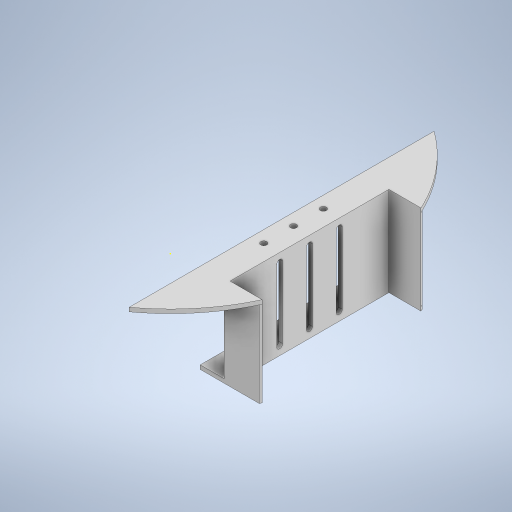
# Autodesk Inventor part: Base-Dribler
Saved by Autodesk Inventor 2024.2 (Build 282272000, 272)
## iProperties
Created: 2023-12-01
Part Number: Base-Dribler
Material: Generic
Document SubType Name: Modeling
Designer: felip
Density: 1 g/cm^3
Appearance: Default
Author: felip
Autodesk Inventor part; units mm, degrees
ref_plane "YZ Plane" through (0, 0, 0) normal (1, 0, 0) x (0, 1, 0)
ref_plane "XZ Plane" through (0, 0, 0) normal (0, 1, 0) x (-1, 0, 0)
ref_plane "XY Plane" through (0, 0, 0) normal (0, 0, 1) x (1, 0, 0)
sketch "Sketch3" plane through (0, 0, 0) normal (0, 1, 0) x (-1, 0, 0)
  circle A0 centre (0, 0) radius 95
  line L0 (-68, 0) -> (-68, -40)
  line L1 (-68, 0) -> (-68, 40)
  line L2 (-68, 40) -> (-86.1684, 40)
  line L3 (-68, -40) -> (-86.1684, -40)
  line L4 (-56, 0) -> (-56, -76.7398)
  line L5 (-56, 0) -> (-56, 76.7398)
  line L6 (-62, 0) -> (-62, -15)
  line L7 (-62, 0) -> (-62, 15)
  circle A1 centre (-62, 15) radius 1.5
  circle A2 centre (-62, 0) radius 1.5
  circle A3 centre (-62, -15) radius 1.5
  line L8 (-68, 0) -> (-70, 0)
  line L9 (-70, 0) -> (-70, -40)
  line L10 (-70, 0) -> (-70, 40)
  dimension "d1" = 68
  dimension "d2" = 40
  dimension "d3" = 40
  dimension "d4" = 12
  dimension "d5" = 6
  dimension "d6" = 15
  dimension "d7" = 15
  dimension "d8" = 3
  dimension "d9" = 3
  dimension "d10" = 3
  dimension "d11" = 2
  constraints: 22 end point, 4 centre point, 4 coincident, 4 point on circle, 4 point on line, 3 vertical, 2 perpendicular, 1 horizontal, 1 parallel
  measures "d1" distance of A0.centre L0.start
  measures "d2" distance of L0.start L0.end
  measures "d3" distance of L0.start L1.end
  measures "d4" distance of L0.start L4.start
  measures "d5" distance of L0.start L6.start
  measures "d6" distance of L6.start L6.end
  measures "d7" distance of L6.start L7.end
  measures "d8" diameter of A1
  measures "d9" diameter of A2
  measures "d10" diameter of A3
  measures "d11" distance of L0.start L8.end
extrude "Extrusion1" add sketch "Sketch3" along normal blind 2 contours L5 L4 A0 L3 L0 L1 L2 | L2 L1 L8 L10 | L9 L8 L0 L3
sketch "Sketch4" plane through (0, 0, 0) normal (0, -1, 0) x (1, 0, 0)
  line L0 (70, 40) -> (70, -40) projected
  line L1 (70, 0) -> (68, 0)
  line L2 (68, 0) -> (68, -40)
  line L3 (70, -41) -> (85.6971, -41)
  arc A0 (56, -76.7398) -> (86.1684, -40) centre (0, 0) ccw projected
  line L4 (68, -40) -> (68, -41)
  line L5 (70, -41) -> (68, -41)
  line L6 (85.6971, -41) -> (86.1684, -40)
  line L7 (70, -40) -> (86.1684, -40) projected
  line L8 (70, -40) -> (86.1684, -40)
  line L9 (70, -40) -> (70, 40)
  line L10 (86.1684, 40) -> (70, 40) projected
  line L11 (86.1684, 40) -> (70, 40)
  line L12 (68, 0) -> (68, 40)
  line L13 (70, 41) -> (85.6971, 41)
  arc A1 (86.1684, 40) -> (56, 76.7398) centre (0, 0) ccw projected
  line L14 (70, 41) -> (68, 41)
  line L15 (68, 40) -> (68, 41)
  line L16 (85.6971, 41) -> (86.1684, 40)
  dimension "d14" = 2
  dimension "d15" = 1
  constraints: 28 end point, 4 point on line, 3 horizontal, 3 perpendicular, 2 point on circle, 1 collinear, 1 midpoint, 1 vertical
  measures "d14" distance of L1.start L1.end
  measures "d15" distance of L0.end L3.start
extrude "Extrusion2" add sketch "Sketch4" along normal blind 41
sketch "Sketch5" plane through (0, -41, 0) normal (0, -1, 0) x (1, 0, 0)
  point P0 (0, 0)
sketch "Sketch6" plane through (0, -41, 0) normal (0, -1, 0) x (1, 0, 0)
  circle A0 centre (62, 15) radius 1.5 projected
  circle A1 centre (62, 15) radius 1.5
  circle A2 centre (62, 0) radius 1.5
  circle A3 centre (62, -15) radius 1.5 projected
  circle A4 centre (62, -15) radius 1.5
  line L0 (70, 40) -> (56, 40)
  line L1 (70, -40) -> (86.1684, -40) projected
  line L2 (70, -40) -> (56, -40)
  line L3 (56, -40) -> (56, 40)
  line L4 (70, 40) -> (70, -40) projected
  line L5 (70, 40) -> (70, -40)
  line L6 (86.1684, 40) -> (70, 40) projected
  line L7 (86.1684, 40) -> (70, 40)
  line L8 (70, -40) -> (86.1684, -40)
  line L9 (86.1684, 40) -> (85.6971, 41)
  arc A5 (86.1684, 40) -> (85.6971, 41) centre (0, 0) ccw projected
  line L10 (56, 40) -> (56, 41)
  line L11 (85.6971, 41) -> (56, 41)
  line L12 (56, -40) -> (56, -41)
  line L13 (86.1684, -40) -> (85.9357, -40.5014)
  line L14 (85.6971, -41) -> (56, -41)
  line L15 (85.9357, -40.5014) -> (85.6971, -41)
  arc A6 (56, -76.7398) -> (86.1684, -40) centre (0, 0) ccw projected
  constraints: 26 end point, 3 centre point, 3 horizontal, 3 perpendicular, 2 coincident, 2 collinear, 2 other
extrude "Extrusion3" add sketch "Sketch6" along normal blind 2 contours L4 L2 L3 L0
extrude "Extrusion5" add sketch "Sketch6" along normal blind 2 contours L0 L10 L11 L9 L6 | L1 L13 L15 L14 L12 L2
sketch "Sketch7" plane through (70, 2, 40) normal (1, 0, 0) x (0, 0, -1)
  line L0 (0, -2) -> (0, -45) projected
  line L1 (80, -2) -> (80, -43) projected
  line L2 (80, -22.5) -> (55, -22.5)
  line L3 (55, -22.5) -> (40, -22.5)
  line L4 (40, -22.5) -> (40, -4.5)
  line L5 (40, -22.5) -> (40, -40.5)
  line L6 (55, -22.5) -> (55, -4.5)
  line L7 (55, -22.5) -> (55, -40.5)
  line L8 (0, 0) -> (80, 0) projected
  line L9 (0, -22.5) -> (25, -22.5)
  line L10 (25, -22.5) -> (25, -4.5)
  line L11 (25, -22.5) -> (25, -40.5)
  line L12 (25, -4.5) -> (25, -40.5) construction
  line L13 (23.5, -4.5) -> (23.5, -40.5)
  line L14 (26.5, -40.5) -> (26.5, -4.5)
  arc A0 (26.5, -4.5) -> (23.5, -4.5) centre (25, -4.5) ccw
  arc A1 (23.5, -40.5) -> (26.5, -40.5) centre (25, -40.5) ccw
  line L15 (40, -4.5) -> (40, -40.5) construction
  line L16 (38.5, -4.5) -> (38.5, -40.5)
  line L17 (41.5, -40.5) -> (41.5, -4.5)
  arc A2 (41.5, -4.5) -> (38.5, -4.5) centre (40, -4.5) ccw
  arc A3 (38.5, -40.5) -> (41.5, -40.5) centre (40, -40.5) ccw
  line L18 (55, -40.5) -> (55, -4.5) construction
  line L19 (56.5, -40.5) -> (56.5, -4.5)
  line L20 (53.5, -4.5) -> (53.5, -40.5)
  arc A4 (53.5, -40.5) -> (56.5, -40.5) centre (55, -40.5) ccw
  arc A5 (56.5, -4.5) -> (53.5, -4.5) centre (55, -4.5) ccw
  point P0 (40, -2)
  dimension "d26" = 25
  dimension "d27" = 15
  dimension "d28" = 18
  dimension "d29" = 18
  dimension "d30" = 18
  dimension "d31" = 18
  dimension "d35" = 22.5
  dimension "d36" = 25
  dimension "d37" = 18
  dimension "d38" = 18
  dimension "d39" = 3
  dimension "d40" = 3
  dimension "d41" = 3
  constraints: 42 end point, 12 point on circle, 12 tangent, 6 centre point, 5 vertical, 4 midpoint, 3 parallel, 2 collinear, 2 horizontal, 2 perpendicular, 2 point on line
  measures "d26" distance of L2.start L2.end
  measures "d27" distance of L2.end L3.end
  measures "d28" distance of L3.end L4.end
  measures "d29" distance of L3.end L5.end
  measures "d30" distance of L2.end L6.end
  measures "d31" distance of L2.end L7.end
  measures "d35" distance between parallel lines of L2 L8
  measures "d36" distance of L9.start L9.end
  measures "d37" distance of L9.end L10.end
  measures "d38" distance of L9.end L11.end
  measures "d39" diameter of A1
  measures "d40" diameter of A3
  measures "d41" diameter of A5
extrude "Extrusion6" cut sketch "Sketch7" against normal blind 2
body "Solid1"
